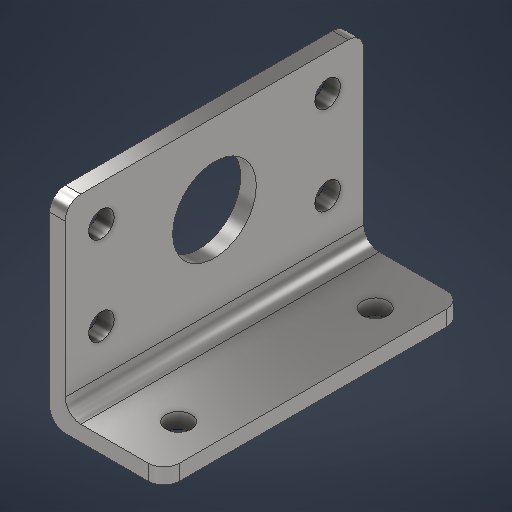
# Autodesk Inventor part: CNC-022-XAxisBallScrewStabilizerMount
Saved by Autodesk Inventor 2026.2 (Build 302298000, 298)
## iProperties
Created: 2026-06-24
Part Number: CNC-022-XAxisBallScrewStabilizerMount
Material: Steel, Mild
Document SubType Name: Modeling
Designer: Kenji
Density: 7.85 g/cm^3
Appearance: Semi-Polished
Author: Kenji
Autodesk Inventor part; units mm, degrees
ref_plane "YZ Plane" through (0, 0, 0) normal (1, 0, 0) x (0, 1, 0)
ref_plane "XZ Plane" through (0, 0, 0) normal (0, 1, 0) x (-1, 0, 0)
ref_plane "XY Plane" through (0, 0, 0) normal (0, 0, 1) x (1, 0, 0)
sketch "Sketch1" plane through (0, 0, 0) normal (1, 0, 0) x (0, 1, 0)
  line L0 (-9, -23) -> (9, -23) construction
  line L1 (9, -23) -> (9, 23) construction
  line L2 (9, 23) -> (-9, 23) construction
  line L3 (-9, 23) -> (-9, -23) construction
  line L4 (-9, -23) -> (9, 23) construction
  line L5 (9, -23) -> (-9, 23) construction
  circle A0 centre (9, 23) radius 2.6
  circle A1 centre (9, -23) radius 2.6
  circle A2 centre (-9, -23) radius 2.6
  circle A3 centre (-9, 23) radius 2.6
  circle A4 centre (9, 23) radius 7.3625 construction
  circle A5 centre (9, -23) radius 7.3625 construction
  circle A6 centre (-9, -23) radius 7.3625 construction
  circle A7 centre (-9, 23) radius 7.3625 construction
  line L6 (16.3625, 30.3625) -> (-21, 30.3625)
  line L7 (-21, 30.3625) -> (-21, -30.3625)
  line L8 (-21, -30.3625) -> (16.3625, -30.3625)
  line L9 (16.3625, -30.3625) -> (16.3625, 30.3625)
  point P0 (0, 0)
  dimension "d0" = 5.2
  dimension "d1" = 46
  dimension "d2" = 18
  dimension "d3" = 4.7625
  dimension "d7" = 12
  constraints: 20 end point, 8 centre point, 7 coincident, 6 equal radius, 4 parallel, 3 tangent, 2 horizontal, 2 midpoint, 2 perpendicular
  measures "d0" diameter of A0
  measures "d1" distance of L0.end L1.end
  measures "d2" distance of L2.end L1.end
  measures "d3" radial gap between concentric circles of A4 A0
  measures "d7" distance from line of L7 L0.start
extrude "Extrusion1" add sketch "Sketch1" along normal blind 3.175
sketch "Sketch3" plane through (0, -21, -30.3625) normal (0, -1, 0) x (1, 0, 0)
  circle A0 centre (15.875, 50.3625) radius 2.6
  line L0 (0, 60.725) -> (0, 0) projected
  circle A1 centre (15.875, 10.3625) radius 2.6
  line L1 (3.175, 60.725) -> (3.175, 0) projected
  circle A2 centre (15.875, 50.3625) radius 7.3625 construction
  circle A3 centre (15.875, 10.3625) radius 7.3625 construction
  line L2 (23.2375, 60.725) -> (0, 60.725)
  line L3 (0, 60.725) -> (0, 0)
  line L4 (0, 0) -> (23.2375, 0)
  line L5 (23.2375, 0) -> (23.2375, 60.725)
  line L6 (0, 60.725) -> (3.175, 60.725) projected
  point P0 (0, 30.3625)
  point P1 (0, 30.3625)
  point P2 (0, 30.3625)
  dimension "d8" = 5.2
  dimension "d9" = 20
  dimension "d10" = 20
  dimension "d11" = 12.7
  dimension "d12" = 4.7625
  constraints: 8 end point, 4 centre point, 2 equal radius, 2 midpoint, 2 parallel, 1 coincident, 1 collinear, 1 horizontal, 1 perpendicular, 1 tangent, 1 vertical alignment
  measures "d8" diameter of A0
  measures "d9" vertical distance of point (0, 30.362) A0.centre
  measures "d10" vertical distance of point (0, 30.362) A1.centre
  measures "d11" distance from line of L1 A1.centre
  measures "d12" radial gap between concentric circles of A2 A0
extrude "Extrusion2" add sketch "Sketch3" along normal blind 3.175
fillet "Fillet1" radius 3.175 2 edges at (3.175, -21, 0) (0, -24.175, 0)
fillet "Fillet2" radius 3.175 4 edges at (1.5875, 16.3625, 30.3625) (1.5875, 16.3625, -30.3625) (23.2375, -22.5875, 30.3625) (23.2375, -22.5875, -30.3625)
sketch "Sketch4" plane through (3.175, 0, 0) normal (1, 0, 0) x (0, 0, -1)
  circle A0 centre (0, 0) radius 8.5
  dimension "d17" = 17
  constraints: 1 centre point, 1 coincident
  measures "d17" diameter of A0
extrude "Extrusion3" cut sketch "Sketch4" against normal through all
equation "\"d10\" = d9"
body "Solid1"
